Autodesk Fusion 360 part; units mm, degrees
note: some values were not read from the file. Set by a fixed rule: which face or edge a step refers to.
(part 2 of 3)
sketch "スケッチ1" plane through (0, 0, 0) normal (0, 0, 1) x (1, 0, 0)
  line L0 (95, 5) -> (-95, 5)
  line L1 (-95, 5) -> (-95, -5)
  line L2 (-95, -5) -> (95, -5)
  line L3 (95, -5) -> (95, 5)
  line L4 (95, 5) -> (-95, -5) construction
  line L5 (-95, 5) -> (95, -5) construction
  line L6 (90, 5) -> (-90, 5)
  line L7 (-90, 5) -> (-90, 25)
  line L8 (-90, 25) -> (90, 25)
  line L9 (90, 25) -> (90, 5)
  line L10 (90, 5) -> (-90, 25) construction
  line L11 (-90, 5) -> (90, 25) construction
  line L12 (90, 25) -> (-90, 25)
  line L13 (-90, 25) -> (-90, 45)
  line L14 (-90, 45) -> (90, 45)
  line L15 (90, 45) -> (90, 25)
  line L16 (90, 25) -> (-90, 45) construction
  line L17 (-90, 25) -> (90, 45) construction
  line L18 (40, -18) -> (-40, -18)
  line L19 (-40, -18) -> (-40, -5)
  line L20 (-40, -5) -> (40, -5)
  line L21 (40, -5) -> (40, -18)
  line L22 (40, -18) -> (-40, -5) construction
  line L23 (-40, -18) -> (40, -5) construction
  point P0 (0, 15)
  point P1 (0, 35)
  point P2 (0, -11.5)
  dimension "d1" = 190
  dimension "d2" = 10
  dimension "d3" = 20
  dimension "d4" = 180
  dimension "d5" = 180
  dimension "d6" = 20
  dimension "d9" = 13
  dimension "d10" = 80
  constraint horizontal L0
  constraint perpendicular L0 L1
  constraint parallel L0 L2
  constraint parallel L1 L3
  constraint coincident L4 origin
  constraint coincident L5 origin
  constraint horizontal L6
  constraint perpendicular L6 L7
  constraint parallel L6 L8
  constraint parallel L7 L9
  constraint coincident L10 P0
  constraint coincident L11 P0
  constraint vertical origin P0
  constraint coincident L0 L6.end
  constraint horizontal L12
  constraint perpendicular L12 L13
  constraint parallel L12 L14
  constraint parallel L13 L15
  constraint coincident L16 P1
  constraint coincident L17 P1
  constraint vertical origin P1
  constraint coincident L8 L7.end
  constraint horizontal L18
  constraint perpendicular L18 L19
  constraint parallel L18 L20
  constraint parallel L19 L21
  constraint coincident L22 P2
  constraint coincident L23 P2
  constraint vertical origin P2
  constraint coincident L2 L19.end
  measures "d1" distance of L1.end L2.end
  measures "d2" distance of L0.end L1.end
  measures "d3" distance of L6.end L7.end
  measures "d4" distance of L7.end L8.end
  measures "d5" distance of L13.end L14.end
  measures "d6" distance of L7.end L13.end
  measures "d9" distance of L18.end L19.end
  measures "d10" distance of L18.start L18.end
extrude "押し出し1" add sketch "スケッチ1" along normal blind 3
sketch "スケッチ2" plane through (0, 0, 0) normal (1, 0, 0) x (0, 1, 0)
  line L0 (-5, 0) -> (-18, 0)
  line L1 (-18, 0) -> (-18, 3)
  line L2 (-18, 3) -> (-5, 3)
  line L3 (-5, 3) -> (-5, 0)
  line L4 (5, 0) -> (-5, 0)
  line L5 (-5, 0) -> (-5, 3)
  line L6 (-5, 3) -> (5, 3)
  line L7 (5, 3) -> (5, 0)
  line L8 (45, 0) -> (5, 0)
  line L9 (5, 0) -> (5, 3)
  line L10 (5, 3) -> (45, 3)
  line L11 (45, 3) -> (45, 0)
  circle A0 centre (-22, 0) radius 2.5
  line L12 (-18, 0) -> (-18, 3)
  line L13 (-18, 0) -> (-19.5, 0)
  line L14 (-18, 3) -> (-24.5, 3)
  line L15 (-24.5, 0) -> (-24.5, 3)
  dimension "d11" = 5
  dimension "d12" = 4
  constraint coincident L0.end L1.start
  constraint coincident A0 L13.end
  constraint perpendicular L1 L13
  constraint coincident L1.end L2.start
  constraint perpendicular L12 L14
  constraint coincident A0 L15.start
  constraint perpendicular L14 L15
  constraint coincident L14.end L15.end
  measures "d11" diameter of A0
  measures "d12" distance of A0.centre L12
extrude "押し出し2" add sketch "スケッチ2" along normal mid plane 80 contours L1 A0 L12 L13 L14 L15 | A0
extrude "押し出し3" add sketch "スケッチ2" along normal mid plane 88 contours A0

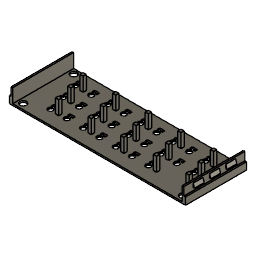
design "Keybord-Base-mid"
Autodesk Fusion 360 part; units mm, degrees
sketch "スケッチ1" plane through (0, 0, 0) normal (0, 0, 1) x (1, 0, 0)
  line L0 (108, 37.5) -> (-108, 37.5)
  line L1 (-108, 37.5) -> (-108, -37.5)
  line L2 (-108, -37.5) -> (108, -37.5)
  line L3 (108, -37.5) -> (108, 37.5)
  line L4 (108, 37.5) -> (-108, -37.5) construction
  line L5 (-108, 37.5) -> (108, -37.5) construction
  line L6 (-3.85, 21.5) -> (-3.85, 24)
  line L7 (-2, 27) -> (-2, 24)
  line L8 (-8, 27) -> (-2, 27)
  line L9 (-2, 24) -> (-8, 24)
  circle A0 centre (-5, 20) radius 2.65
  line L10 (-8, 24) -> (-8, 27)
  line L11 (-6.15, 24) -> (-6.15, 21.5)
  line L12 (-6.15, 21.5) -> (-3.85, 21.5)
  line L13 (-8, 24) -> (-2, 27) construction
  line L14 (-2, 24) -> (-8, 27) construction
  line L15 (-5, 20) -> (-5, 34)
  line L16 (-85, 20) -> (-85, 34)
  line L17 (-88, 24) -> (-88, 27)
  line L18 (-83.85, 21.5) -> (-83.85, 24)
  line L19 (-88, 24) -> (-82, 27) construction
  line L20 (-82, 27) -> (-82, 24)
  line L21 (-88, 27) -> (-82, 27)
  line L22 (-82, 24) -> (-88, 27) construction
  circle A1 centre (-85, 20) radius 2.65
  line L23 (-86.15, 24) -> (-86.15, 21.5)
  line L24 (-86.15, 21.5) -> (-83.85, 21.5)
  line L25 (-82, 24) -> (-88, 24)
  line L26 (-65, 20) -> (-65, 34)
  line L27 (-68, 24) -> (-68, 27)
  line L28 (-63.85, 21.5) -> (-63.85, 24)
  line L29 (-68, 24) -> (-62, 27) construction
  line L30 (-62, 27) -> (-62, 24)
  line L31 (-68, 27) -> (-62, 27)
  line L32 (-62, 24) -> (-68, 27) construction
  circle A2 centre (-65, 20) radius 2.65
  line L33 (-66.15, 24) -> (-66.15, 21.5)
  line L34 (-66.15, 21.5) -> (-63.85, 21.5)
  line L35 (-62, 24) -> (-68, 24)
  line L36 (-45, 20) -> (-45, 34)
  line L37 (-48, 24) -> (-48, 27)
  line L38 (-43.85, 21.5) -> (-43.85, 24)
  line L39 (-48, 24) -> (-42, 27) construction
  line L40 (-42, 27) -> (-42, 24)
  line L41 (-48, 27) -> (-42, 27)
  line L42 (-42, 24) -> (-48, 27) construction
  circle A3 centre (-45, 20) radius 2.65
  line L43 (-46.15, 24) -> (-46.15, 21.5)
  line L44 (-46.15, 21.5) -> (-43.85, 21.5)
  line L45 (-42, 24) -> (-48, 24)
  line L46 (-25, 20) -> (-25, 34)
  line L47 (-28, 24) -> (-28, 27)
  line L48 (-23.85, 21.5) -> (-23.85, 24)
  line L49 (-28, 24) -> (-22, 27) construction
  line L50 (-22, 27) -> (-22, 24)
  line L51 (-28, 27) -> (-22, 27)
  line L52 (-22, 24) -> (-28, 27) construction
  circle A4 centre (-25, 20) radius 2.65
  line L53 (-26.15, 24) -> (-26.15, 21.5)
  line L54 (-26.15, 21.5) -> (-23.85, 21.5)
  line L55 (-22, 24) -> (-28, 24)
  line L56 (15, 20) -> (15, 34)
  line L57 (12, 24) -> (12, 27)
  line L58 (16.15, 21.5) -> (16.15, 24)
  line L59 (12, 24) -> (18, 27) construction
  line L60 (18, 27) -> (18, 24)
  line L61 (12, 27) -> (18, 27)
  line L62 (18, 24) -> (12, 27) construction
  circle A5 centre (15, 20) radius 2.65
  line L63 (13.85, 24) -> (13.85, 21.5)
  line L64 (13.85, 21.5) -> (16.15, 21.5)
  line L65 (18, 24) -> (12, 24)
  line L66 (35, 20) -> (35, 34)
  line L67 (32, 24) -> (32, 27)
  line L68 (36.15, 21.5) -> (36.15, 24)
  line L69 (32, 24) -> (38, 27) construction
  line L70 (38, 27) -> (38, 24)
  line L71 (32, 27) -> (38, 27)
  line L72 (38, 24) -> (32, 27) construction
  circle A6 centre (35, 20) radius 2.65
  line L73 (33.85, 24) -> (33.85, 21.5)
  line L74 (33.85, 21.5) -> (36.15, 21.5)
  line L75 (38, 24) -> (32, 24)
  line L76 (55, 20) -> (55, 34)
  line L77 (52, 24) -> (52, 27)
  line L78 (56.15, 21.5) -> (56.15, 24)
  line L79 (52, 24) -> (58, 27) construction
  line L80 (58, 27) -> (58, 24)
  line L81 (52, 27) -> (58, 27)
  line L82 (58, 24) -> (52, 27) construction
  circle A7 centre (55, 20) radius 2.65
  line L83 (53.85, 24) -> (53.85, 21.5)
  line L84 (53.85, 21.5) -> (56.15, 21.5)
  line L85 (58, 24) -> (52, 24)
  line L86 (75, 20) -> (75, 34)
  line L87 (72, 24) -> (72, 27)
  line L88 (76.15, 21.5) -> (76.15, 24)
  line L89 (72, 24) -> (78, 27) construction
  line L90 (78, 27) -> (78, 24)
  line L91 (72, 27) -> (78, 27)
  line L92 (78, 24) -> (72, 27) construction
  circle A8 centre (75, 20) radius 2.65
  line L93 (73.85, 24) -> (73.85, 21.5)
  line L94 (73.85, 21.5) -> (76.15, 21.5)
  line L95 (78, 24) -> (72, 24)
  line L96 (95, 20) -> (95, 34)
  line L97 (92, 24) -> (92, 27)
  line L98 (96.15, 21.5) -> (96.15, 24)
  line L99 (92, 24) -> (98, 27) construction
  line L100 (98, 27) -> (98, 24)
  line L101 (92, 27) -> (98, 27)
  line L102 (98, 24) -> (92, 27) construction
  circle A9 centre (95, 20) radius 2.65
  line L103 (93.85, 24) -> (93.85, 21.5)
  line L104 (93.85, 21.5) -> (96.15, 21.5)
  line L105 (98, 24) -> (92, 24)
  line L106 (-3, 4) -> (-3, 7)
  line L107 (0, 0) -> (0, 14)
  line L108 (1.15, 1.5) -> (1.15, 4)
  line L109 (-3, 7) -> (3, 7)
  line L110 (-1.15, 1.5) -> (1.15, 1.5)
  line L111 (3, 7) -> (3, 4)
  line L112 (-3, 4) -> (3, 7) construction
  circle A10 centre (0, 0) radius 2.65
  line L113 (3, 4) -> (-3, 7) construction
  line L114 (3, 4) -> (-3, 4)
  line L115 (-1.15, 4) -> (-1.15, 1.5)
  circle A11 centre (-80, 0) radius 2.65
  line L116 (-83, 4) -> (-83, 7)
  line L117 (-83, 7) -> (-77, 7)
  line L118 (-77, 4) -> (-83, 4)
  line L119 (-77, 7) -> (-77, 4)
  line L120 (-82.2732, 4.8091) -> (-76.2732, 7.8091) construction
  line L121 (-76.2732, 4.8091) -> (-82.2732, 7.8091) construction
  line L122 (-81.15, 4) -> (-81.15, 1.5)
  line L123 (-81.15, 1.5) -> (-78.85, 1.5)
  line L124 (-78.85, 1.5) -> (-78.85, 4)
  circle A12 centre (-60, 0) radius 2.65
  line L125 (-63, 4) -> (-63, 7)
  line L126 (-63, 7) -> (-57, 7)
  line L127 (-57, 4) -> (-63, 4)
  line L128 (-57, 7) -> (-57, 4)
  line L129 (-62.2732, 4.8091) -> (-56.2732, 7.8091) construction
  line L130 (-56.2732, 4.8091) -> (-62.2732, 7.8091) construction
  line L131 (-61.15, 4) -> (-61.15, 1.5)
  line L132 (-61.15, 1.5) -> (-58.85, 1.5)
  line L133 (-58.85, 1.5) -> (-58.85, 4)
  circle A13 centre (-40, 0) radius 2.65
  line L134 (-43, 4) -> (-43, 7)
  line L135 (-43, 7) -> (-37, 7)
  line L136 (-37, 4) -> (-43, 4)
  line L137 (-37, 7) -> (-37, 4)
  line L138 (-42.2732, 4.8091) -> (-36.2732, 7.8091) construction
  line L139 (-36.2732, 4.8091) -> (-42.2732, 7.8091) construction
  line L140 (-41.15, 4) -> (-41.15, 1.5)
  line L141 (-41.15, 1.5) -> (-38.85, 1.5)
  line L142 (-38.85, 1.5) -> (-38.85, 4)
  circle A14 centre (-20, 0) radius 2.65
  line L143 (-23, 4) -> (-23, 7)
  line L144 (-23, 7) -> (-17, 7)
  line L145 (-17, 4) -> (-23, 4)
  line L146 (-17, 7) -> (-17, 4)
  line L147 (-22.2732, 4.8091) -> (-16.2732, 7.8091) construction
  line L148 (-16.2732, 4.8091) -> (-22.2732, 7.8091) construction
  line L149 (-21.15, 4) -> (-21.15, 1.5)
  line L150 (-21.15, 1.5) -> (-18.85, 1.5)
  line L151 (-18.85, 1.5) -> (-18.85, 4)
  circle A15 centre (20, 0) radius 2.65
  line L152 (17, 4) -> (17, 7)
  line L153 (17, 7) -> (23, 7)
  line L154 (23, 4) -> (17, 4)
  line L155 (23, 7) -> (23, 4)
  line L156 (17.7268, 4.8091) -> (23.7268, 7.8091) construction
  line L157 (23.7268, 4.8091) -> (17.7268, 7.8091) construction
  line L158 (18.85, 4) -> (18.85, 1.5)
  line L159 (18.85, 1.5) -> (21.15, 1.5)
  line L160 (21.15, 1.5) -> (21.15, 4)
  circle A16 centre (40, 0) radius 2.65
  line L161 (37, 4) -> (37, 7)
  line L162 (37, 7) -> (43, 7)
  line L163 (43, 4) -> (37, 4)
  line L164 (43, 7) -> (43, 4)
  line L165 (37.7268, 4.8091) -> (43.7268, 7.8091) construction
  line L166 (43.7268, 4.8091) -> (37.7268, 7.8091) construction
  line L167 (38.85, 4) -> (38.85, 1.5)
  line L168 (38.85, 1.5) -> (41.15, 1.5)
  line L169 (41.15, 1.5) -> (41.15, 4)
  circle A17 centre (60, 0) radius 2.65
  line L170 (57, 4) -> (57, 7)
  line L171 (57, 7) -> (63, 7)
  line L172 (63, 4) -> (57, 4)
  line L173 (63, 7) -> (63, 4)
  line L174 (57.7268, 4.8091) -> (63.7268, 7.8091) construction
  line L175 (63.7268, 4.8091) -> (57.7268, 7.8091) construction
  line L176 (58.85, 4) -> (58.85, 1.5)
  line L177 (58.85, 1.5) -> (61.15, 1.5)
  line L178 (61.15, 1.5) -> (61.15, 4)
  circle A18 centre (80, 0) radius 2.65
  line L179 (77, 4) -> (77, 7)
  line L180 (77, 7) -> (83, 7)
  line L181 (83, 4) -> (77, 4)
  line L182 (83, 7) -> (83, 4)
  line L183 (77.7268, 4.8091) -> (83.7268, 7.8091) construction
  line L184 (83.7268, 4.8091) -> (77.7268, 7.8091) construction
  line L185 (78.85, 4) -> (78.85, 1.5)
  line L186 (78.85, 1.5) -> (81.15, 1.5)
  line L187 (81.15, 1.5) -> (81.15, 4)
  line L188 (8, -16) -> (2, -13) construction
  line L189 (5, -20) -> (5, -6)
  line L190 (3.85, -18.5) -> (6.15, -18.5)
  line L191 (2, -13) -> (8, -13)
  line L192 (2, -16) -> (2, -13)
  line L193 (2, -16) -> (8, -13) construction
  line L194 (8, -13) -> (8, -16)
  circle A19 centre (5, -20) radius 2.65
  line L195 (3.85, -16) -> (3.85, -18.5)
  line L196 (6.15, -18.5) -> (6.15, -16)
  line L197 (8, -16) -> (2, -16)
  circle A20 centre (45, -20) radius 2.65
  line L198 (45, -20) -> (45, -6)
  line L199 (46.15, -18.5) -> (46.15, -16)
  line L200 (43.85, -18.5) -> (46.15, -18.5)
  line L201 (48, -16) -> (42, -16)
  line L202 (43.85, -16) -> (43.85, -18.5)
  line L203 (48, -16) -> (42, -13) construction
  line L204 (42, -16) -> (48, -13) construction
  line L205 (42, -13) -> (48, -13)
  line L206 (42, -16) -> (42, -13)
  line L207 (48, -13) -> (48, -16)
  circle A21 centre (25, -20) radius 2.65
  line L208 (25, -20) -> (25, -6)
  line L209 (26.15, -18.5) -> (26.15, -16)
  line L210 (23.85, -18.5) -> (26.15, -18.5)
  line L211 (28, -16) -> (22, -16)
  line L212 (23.85, -16) -> (23.85, -18.5)
  line L213 (28, -16) -> (22, -13) construction
  line L214 (22, -16) -> (28, -13) construction
  line L215 (22, -13) -> (28, -13)
  line L216 (22, -16) -> (22, -13)
  line L217 (28, -13) -> (28, -16)
  circle A22 centre (-15, -20) radius 2.65
  line L218 (-15, -20) -> (-15, -6)
  line L219 (-13.85, -18.5) -> (-13.85, -16)
  line L220 (-16.15, -18.5) -> (-13.85, -18.5)
  line L221 (-12, -16) -> (-18, -16)
  line L222 (-16.15, -16) -> (-16.15, -18.5)
  line L223 (-12, -16) -> (-18, -13) construction
  line L224 (-18, -16) -> (-12, -13) construction
  line L225 (-18, -13) -> (-12, -13)
  line L226 (-18, -16) -> (-18, -13)
  line L227 (-12, -13) -> (-12, -16)
  circle A23 centre (-35, -20) radius 2.65
  line L228 (-35, -20) -> (-35, -6)
  line L229 (-33.85, -18.5) -> (-33.85, -16)
  line L230 (-36.15, -18.5) -> (-33.85, -18.5)
  line L231 (-32, -16) -> (-38, -16)
  line L232 (-36.15, -16) -> (-36.15, -18.5)
  line L233 (-32, -16) -> (-38, -13) construction
  line L234 (-38, -16) -> (-32, -13) construction
  line L235 (-38, -13) -> (-32, -13)
  line L236 (-38, -16) -> (-38, -13)
  line L237 (-32, -13) -> (-32, -16)
  circle A24 centre (-55, -20) radius 2.65
  line L238 (-55, -20) -> (-55, -6)
  line L239 (-53.85, -18.5) -> (-53.85, -16)
  line L240 (-56.15, -18.5) -> (-53.85, -18.5)
  line L241 (-52, -16) -> (-58, -16)
  line L242 (-56.15, -16) -> (-56.15, -18.5)
  line L243 (-52, -16) -> (-58, -13) construction
  line L244 (-58, -16) -> (-52, -13) construction
  line L245 (-58, -13) -> (-52, -13)
  line L246 (-58, -16) -> (-58, -13)
  line L247 (-52, -13) -> (-52, -16)
  circle A25 centre (-75, -20) radius 2.65
  line L248 (-75, -20) -> (-75, -6)
  line L249 (-73.85, -18.5) -> (-73.85, -16)
  line L250 (-76.15, -18.5) -> (-73.85, -18.5)
  line L251 (-72, -16) -> (-78, -16)
  line L252 (-76.15, -16) -> (-76.15, -18.5)
  line L253 (-72, -16) -> (-78, -13) construction
  line L254 (-78, -16) -> (-72, -13) construction
  line L255 (-78, -13) -> (-72, -13)
  line L256 (-78, -16) -> (-78, -13)
  line L257 (-72, -13) -> (-72, -16)
  point P0 (0, 2.65)
  point P1 (-5, 25.5)
  point P2 (-5, 20)
  point P3 (-5, 20)
  point P4 (-5, 22.65)
  point P5 (-85, 22.65)
  point P6 (-85, 25.5)
  point P7 (-85, 20)
  point P8 (-85, 20)
  point P9 (-65, 22.65)
  point P10 (-65, 25.5)
  point P11 (-65, 20)
  point P12 (-65, 20)
  point P13 (-45, 22.65)
  point P14 (-45, 25.5)
  point P15 (-45, 20)
  point P16 (-45, 20)
  point P17 (-25, 22.65)
  point P18 (-25, 25.5)
  point P19 (-25, 20)
  point P20 (-25, 20)
  point P21 (15, 22.65)
  point P22 (15, 25.5)
  point P23 (15, 20)
  point P24 (15, 20)
  point P25 (35, 22.65)
  point P26 (35, 25.5)
  point P27 (35, 20)
  point P28 (35, 20)
  point P29 (55, 22.65)
  point P30 (55, 25.5)
  point P31 (55, 20)
  point P32 (55, 20)
  point P33 (75, 22.65)
  point P34 (75, 25.5)
  point P35 (75, 20)
  point P36 (75, 20)
  point P37 (95, 22.65)
  point P38 (95, 25.5)
  point P39 (95, 20)
  point P40 (95, 20)
  point P41 (-10.2565, 1.2142)
  point P42 (-10.2565, 1.2142)
  point P43 (0, 5.5)
  point P44 (0, 2.65)
  point P45 (5, -20)
  point P46 (5, -17.35)
  point P47 (5, -14.5)
  point P48 (5, -20)
  point P49 (45, -17.35)
  point P50 (45, -20)
  point P51 (45, -20)
  point P52 (45, -14.5)
  point P53 (25, -17.35)
  point P54 (25, -20)
  point P55 (25, -20)
  point P56 (25, -14.5)
  point P57 (-15, -17.35)
  point P58 (-15, -20)
  point P59 (-15, -20)
  point P60 (-15, -14.5)
  point P61 (-35, -17.35)
  point P62 (-35, -20)
  point P63 (-35, -20)
  point P64 (-35, -14.5)
  point P65 (-55, -17.35)
  point P66 (-55, -20)
  point P67 (-55, -20)
  point P68 (-55, -14.5)
  point P69 (-75, -17.35)
  point P70 (-75, -20)
  point P71 (-75, -20)
  point P72 (-75, -14.5)
  dimension "d1" = 216
  dimension "d2" = 75
  dimension "d85" = 5.3
  dimension "d86" = 2.3
  dimension "d87" = 6
  dimension "d88" = 3
  dimension "d89" = 5.5
  dimension "d90" = 1.5
  dimension "d92" = 20
  dimension "d94" = 2.3
  dimension "d97" = 20
  dimension "d98" = 0
  dimension "d99" = 5
  dimension "d114" = 5.3
  dimension "d115" = 2.3
  dimension "d116" = 6
  dimension "d117" = 3
  dimension "d118" = 5.5
  dimension "d119" = 1.5
  dimension "d120" = 2.3
  dimension "d138" = 5.3
  dimension "d139" = 2.3
  dimension "d140" = 6
  dimension "d141" = 3
  dimension "d142" = 5.5
  dimension "d143" = 1.5
  dimension "d144" = 2.3
  dimension "d145" = 5
  dimension "d146" = 20
  dimension "d149" = -20
  dimension "d150" = 0
  constraint horizontal L0
  constraint perpendicular L0 L1
  constraint parallel L0 L2
  constraint parallel L1 L3
  constraint coincident L4 L107.start
  constraint coincident L5 L107.start
  constraint coincident L107.start A10.centre
  constraint vertical L107.start P44
  constraint coincident P3 P2
  constraint parallel L6 L11
  constraint coincident P4 A0
  constraint vertical P3 P4
  constraint horizontal L9
  constraint perpendicular L9 L10
  constraint parallel L8 L9
  constraint parallel L7 L10
  constraint coincident P1 L14
  constraint coincident P1 L13
  constraint perpendicular L11 L12
  constraint coincident L11.start L9
  constraint coincident L6.end L9
  constraint perpendicular L8 L15
  constraint midpoint L8 L15
  constraint coincident P42 P41
  constraint parallel L108 L115
  constraint coincident P44 A10
  constraint horizontal L114
  constraint perpendicular L106 L114
  constraint parallel L109 L114
  constraint parallel L106 L111
  constraint coincident P43 L113
  constraint coincident P43 L112
  constraint perpendicular L110 L115
  constraint coincident L115.start L114
  constraint coincident L108.end L114
  constraint perpendicular L107 L109
  constraint midpoint L107 L109
  constraint coincident P48 P45
  constraint parallel L195 L196
  constraint coincident P46 A19
  constraint vertical P48 P46
  constraint horizontal L197
  constraint perpendicular L192 L197
  constraint parallel L191 L197
  constraint parallel L192 L194
  constraint coincident P47 L188
  constraint coincident P47 L193
  constraint perpendicular L190 L195
  constraint coincident L195.start L197
  constraint coincident L196.end L197
  constraint perpendicular L189 L191
  constraint midpoint L189 L191
  measures "d1" distance of L1.end L2.end
  measures "d2" distance of L0.end L1.end
  measures "d85" diameter of A0
  measures "d86" distance of L11.end L6.start
  measures "d87" distance of L7.start L8.start
  measures "d88" distance of L9.end L8.start
  measures "d89" distance of P1 P3
  measures "d90" distance of P3 L12
  measures "d92" vertical distance of L107.start P3
  measures "d99" horizontal distance of L107.start P3
  measures "d114" diameter of A10
  measures "d115" distance of L110.start L108.start
  measures "d116" distance of L106.end L109.end
  measures "d117" distance of L106.end L106.start
  measures "d118" distance of P43 L107.start
  measures "d119" distance of L107.start L110
  measures "d138" diameter of A19
  measures "d139" distance of L190.start L190.end
  measures "d140" distance of L188.end L191.end
  measures "d141" distance of L188.end L192.start
  measures "d142" distance of P48 P47
  measures "d143" distance of P48 L190
  measures "d145" horizontal distance of L107.start P48
  measures "d146" vertical distance of L107.start P48
extrude "押し出し1" add sketch "スケッチ1" along normal blind 2
fillet "フィレット1" radius 0.5 52 faces at (94.3639, 17.4275, 1.3333) (97.1025, 21.6131, 1.3333) (74.3639, 17.4275, 1.3333) (77.1025, 21.6131, 1.3333) (57.6468, 19.8702, 1.3333) (57.1025, 21.6131, 1.3333) (37.6468, 19.8702, 1.3333) (37.1025, 21.6131, 1.3333) (17.6468, 19.8702, 1.3333) (16.2603, 22.3311, 1.3333) (-2.3532, 19.8702, 1.3333) (-3.7397, 22.3311, 1.3333) (21.5738, 2.1321, 1.3333) (22.6468, -0.1298, 1.3333) (-22.3532, 19.8702, 1.3333) (-22.5332, 20.9681, 1.3333) (-42.3532, 19.8702, 1.3333) (-42.8975, 21.6131, 1.3333) (-65.6361, 17.4275, 1.3333) (-62.8975, 21.6131, 1.3333) (-85.6361, 17.4275, 1.3333) (-82.8975, 21.6131, 1.3333) (-78.6321, 2.2697, 1.3333) (-80.6361, -2.5725, 1.3333) (-58.4262, 2.1321, 1.3333) (-57.3532, -0.1298, 1.3333) (-38.4262, 2.1321, 1.3333) (-37.3532, -0.1298, 1.3333) (-18.1437, 1.8912, 1.3333) (-17.3532, -0.1298, 1.3333) (2.6468, -0.1298, 1.3333) (1.2603, 2.3311, 1.3333) (7.6468, -20.1298, 1.3333) (7.4668, -19.0319, 1.3333) (-12.5332, -19.0319, 1.3333) (-12.3532, -20.1298, 1.3333) (-32.8975, -18.3869, 1.3333) (-32.3532, -20.1298, 1.3333) (-72.8975, -18.3869, 1.3333) (-75.6361, -22.5725, 1.3333) (-52.8975, -18.3869, 1.3333) (-52.3532, -20.1298, 1.3333) (41.5738, 2.1321, 1.3333) (42.6468, -0.1298, 1.3333) (27.4668, -19.0319, 1.3333) (27.6468, -20.1298, 1.3333) (47.1025, -18.3869, 1.3333) (47.6468, -20.1298, 1.3333) (61.5738, 2.1321, 1.3333) (62.6468, -0.1298, 1.3333) (81.3679, 2.2697, 1.3333) (79.3639, -2.5725, 1.3333)
sketch "スケッチ2" plane through (0, 0, 2) normal (0, 0, 1) x (-1, 0, 0)
  line L0 (-108, 37.5) -> (-108, -37.5)
  line L1 (-108, -37.5) -> (108, -37.5)
  line L2 (108, -37.5) -> (108, 37.5)
  line L3 (108, 37.5) -> (-108, 37.5)
  line L4 (108, -37.5) -> (104, -37.5)
  line L5 (104, -37.5) -> (104, 37.5)
  line L6 (104, 37.5) -> (108, 37.5)
  line L7 (108, 37.5) -> (108, -37.5)
  line L8 (-108, -37.5) -> (-104, -37.5)
  line L9 (-104, -37.5) -> (-104, 37.5)
  line L10 (-104, 37.5) -> (-108, 37.5)
  line L11 (-108, 37.5) -> (-108, -37.5)
  line L12 (-18.85, -2.9326) -> (-18.85, -4)
  line L13 (-18.85, -4) -> (-17, -4)
  line L14 (-17, -4) -> (-17, -7)
  line L15 (-17, -7) -> (-23, -7)
  line L16 (-23, -7) -> (-23, -4)
  line L17 (-23, -4) -> (-21.15, -4)
  line L18 (-21.15, -4) -> (-21.15, -2.9326)
  line L19 (16.15, 17.0674) -> (16.15, 16)
  line L20 (16.15, 16) -> (18, 16)
  line L21 (18, 16) -> (18, 13)
  line L22 (18, 13) -> (12, 13)
  line L23 (12, 13) -> (12, 16)
  line L24 (12, 16) -> (13.85, 16)
  line L25 (13.85, 16) -> (13.85, 17.0674)
  line L26 (76.15, 17.0674) -> (76.15, 16)
  line L27 (76.15, 16) -> (78, 16)
  line L28 (78, 16) -> (78, 13)
  line L29 (78, 13) -> (72, 13)
  line L30 (72, 13) -> (72, 16)
  line L31 (72, 16) -> (73.85, 16)
  line L32 (73.85, 16) -> (73.85, 17.0674)
  line L33 (-38.85, -2.9326) -> (-38.85, -4)
  line L34 (-38.85, -4) -> (-37, -4)
  line L35 (-37, -4) -> (-37, -7)
  line L36 (-37, -7) -> (-43, -7)
  line L37 (-43, -7) -> (-43, -4)
  line L38 (-43, -4) -> (-41.15, -4)
  line L39 (-41.15, -4) -> (-41.15, -2.9326)
  line L40 (-43.85, 17.0674) -> (-43.85, 16)
  line L41 (-43.85, 16) -> (-42, 16)
  line L42 (-42, 16) -> (-42, 13)
  line L43 (-42, 13) -> (-48, 13)
  line L44 (-48, 13) -> (-48, 16)
  line L45 (-48, 16) -> (-46.15, 16)
  line L46 (-46.15, 16) -> (-46.15, 17.0674)
  line L47 (-23.85, 17.0674) -> (-23.85, 16)
  line L48 (-23.85, 16) -> (-22, 16)
  line L49 (-22, 16) -> (-22, 13)
  line L50 (-22, 13) -> (-28, 13)
  line L51 (-28, 13) -> (-28, 16)
  line L52 (-28, 16) -> (-26.15, 16)
  line L53 (-26.15, 16) -> (-26.15, 17.0674)
  line L54 (1.15, -4) -> (3, -4)
  line L55 (3, -4) -> (3, -7)
  line L56 (3, -7) -> (-3, -7)
  line L57 (-3, -7) -> (-3, -4)
  line L58 (-3, -4) -> (-1.15, -4)
  line L59 (-1.15, -4) -> (-1.15, -2.9326)
  line L60 (1.15, -2.9326) -> (1.15, -4)
  line L61 (61.15, -2.9326) -> (61.15, -4)
  line L62 (61.15, -4) -> (63, -4)
  line L63 (63, -4) -> (63, -7)
  line L64 (63, -7) -> (57, -7)
  line L65 (57, -7) -> (57, -4)
  line L66 (57, -4) -> (58.85, -4)
  line L67 (58.85, -4) -> (58.85, -2.9326)
  line L68 (56.15, 17.0674) -> (56.15, 16)
  line L69 (56.15, 16) -> (58, 16)
  line L70 (58, 16) -> (58, 13)
  line L71 (58, 13) -> (52, 13)
  line L72 (52, 13) -> (52, 16)
  line L73 (52, 16) -> (53.85, 16)
  line L74 (53.85, 16) -> (53.85, 17.0674)
  line L75 (36.15, 17.0674) -> (36.15, 16)
  line L76 (36.15, 16) -> (38, 16)
  line L77 (38, 16) -> (38, 13)
  line L78 (38, 13) -> (32, 13)
  line L79 (32, 13) -> (32, 16)
  line L80 (32, 16) -> (33.85, 16)
  line L81 (33.85, 16) -> (33.85, 17.0674)
  line L82 (-3.85, 17.0674) -> (-3.85, 16)
  line L83 (-3.85, 16) -> (-2, 16)
  line L84 (-2, 16) -> (-2, 13)
  line L85 (-2, 13) -> (-8, 13)
  line L86 (-8, 13) -> (-8, 16)
  line L87 (-8, 16) -> (-6.15, 16)
  line L88 (-6.15, 16) -> (-6.15, 17.0674)
  line L89 (-58.85, -2.9326) -> (-58.85, -4)
  line L90 (-58.85, -4) -> (-57, -4)
  line L91 (-57, -4) -> (-57, -7)
  line L92 (-57, -7) -> (-63, -7)
  line L93 (-63, -7) -> (-63, -4)
  line L94 (-63, -4) -> (-61.15, -4)
  line L95 (-61.15, -4) -> (-61.15, -2.9326)
  line L96 (81.15, -2.9326) -> (81.15, -4)
  line L97 (81.15, -4) -> (83, -4)
  line L98 (83, -4) -> (83, -7)
  line L99 (83, -7) -> (77, -7)
  line L100 (77, -7) -> (77, -4)
  line L101 (77, -4) -> (78.85, -4)
  line L102 (78.85, -4) -> (78.85, -2.9326)
  line L103 (21.15, -2.9326) -> (21.15, -4)
  line L104 (21.15, -4) -> (23, -4)
  line L105 (23, -4) -> (23, -7)
  line L106 (23, -7) -> (17, -7)
  line L107 (17, -7) -> (17, -4)
  line L108 (17, -4) -> (18.85, -4)
  line L109 (18.85, -4) -> (18.85, -2.9326)
  line L110 (-78.85, -2.9326) -> (-78.85, -4)
  line L111 (-78.85, -4) -> (-77, -4)
  line L112 (-77, -4) -> (-77, -7)
  line L113 (-77, -7) -> (-83, -7)
  line L114 (-83, -7) -> (-83, -4)
  line L115 (-83, -4) -> (-81.15, -4)
  line L116 (-81.15, -4) -> (-81.15, -2.9326)
  line L117 (41.15, -2.9326) -> (41.15, -4)
  line L118 (41.15, -4) -> (43, -4)
  line L119 (43, -4) -> (43, -7)
  line L120 (43, -7) -> (37, -7)
  line L121 (37, -7) -> (37, -4)
  line L122 (37, -4) -> (38.85, -4)
  line L123 (38.85, -4) -> (38.85, -2.9326)
  line L124 (-93.85, -22.9326) -> (-93.85, -24)
  line L125 (-93.85, -24) -> (-92, -24)
  line L126 (-92, -24) -> (-92, -27)
  line L127 (-92, -27) -> (-98, -27)
  line L128 (-98, -27) -> (-98, -24)
  line L129 (-98, -24) -> (-96.15, -24)
  line L130 (-96.15, -24) -> (-96.15, -22.9326)
  line L131 (26.15, -22.9326) -> (26.15, -24)
  line L132 (26.15, -24) -> (28, -24)
  line L133 (28, -24) -> (28, -27)
  line L134 (28, -27) -> (22, -27)
  line L135 (22, -27) -> (22, -24)
  line L136 (22, -24) -> (23.85, -24)
  line L137 (23.85, -24) -> (23.85, -22.9326)
  line L138 (46.15, -22.9326) -> (46.15, -24)
  line L139 (46.15, -24) -> (48, -24)
  line L140 (48, -24) -> (48, -27)
  line L141 (48, -27) -> (42, -27)
  line L142 (42, -27) -> (42, -24)
  line L143 (42, -24) -> (43.85, -24)
  line L144 (43.85, -24) -> (43.85, -22.9326)
  line L145 (6.15, -24) -> (8, -24)
  line L146 (8, -24) -> (8, -27)
  line L147 (8, -27) -> (2, -27)
  line L148 (2, -27) -> (2, -24)
  line L149 (2, -24) -> (3.85, -24)
  line L150 (3.85, -24) -> (3.85, -22.9326)
  line L151 (6.15, -22.9326) -> (6.15, -24)
  line L152 (66.15, -22.9326) -> (66.15, -24)
  line L153 (66.15, -24) -> (68, -24)
  line L154 (68, -24) -> (68, -27)
  line L155 (68, -27) -> (62, -27)
  line L156 (62, -27) -> (62, -24)
  line L157 (62, -24) -> (63.85, -24)
  line L158 (63.85, -24) -> (63.85, -22.9326)
  line L159 (86.15, -22.9326) -> (86.15, -24)
  line L160 (86.15, -24) -> (88, -24)
  line L161 (88, -24) -> (88, -27)
  line L162 (88, -27) -> (82, -27)
  line L163 (82, -27) -> (82, -24)
  line L164 (82, -24) -> (83.85, -24)
  line L165 (83.85, -24) -> (83.85, -22.9326)
  line L166 (-13.85, -22.9326) -> (-13.85, -24)
  line L167 (-13.85, -24) -> (-12, -24)
  line L168 (-12, -24) -> (-12, -27)
  line L169 (-12, -27) -> (-18, -27)
  line L170 (-18, -27) -> (-18, -24)
  line L171 (-18, -24) -> (-16.15, -24)
  line L172 (-16.15, -24) -> (-16.15, -22.9326)
  line L173 (-53.85, -22.9326) -> (-53.85, -24)
  line L174 (-53.85, -24) -> (-52, -24)
  line L175 (-52, -24) -> (-52, -27)
  line L176 (-52, -27) -> (-58, -27)
  line L177 (-58, -27) -> (-58, -24)
  line L178 (-58, -24) -> (-56.15, -24)
  line L179 (-56.15, -24) -> (-56.15, -22.9326)
  line L180 (-33.85, -22.9326) -> (-33.85, -24)
  line L181 (-33.85, -24) -> (-32, -24)
  line L182 (-32, -24) -> (-32, -27)
  line L183 (-32, -27) -> (-38, -27)
  line L184 (-38, -27) -> (-38, -24)
  line L185 (-38, -24) -> (-36.15, -24)
  line L186 (-36.15, -24) -> (-36.15, -22.9326)
  line L187 (-73.85, -22.9326) -> (-73.85, -24)
  line L188 (-73.85, -24) -> (-72, -24)
  line L189 (-72, -24) -> (-72, -27)
  line L190 (-72, -27) -> (-78, -27)
  line L191 (-78, -27) -> (-78, -24)
  line L192 (-78, -24) -> (-76.15, -24)
  line L193 (-76.15, -24) -> (-76.15, -22.9326)
  arc A0 (-78.85, -2.9326) -> (-81.15, -2.9326) centre (-80, 0) ccw
  arc A1 (-58.85, -2.9326) -> (-61.15, -2.9326) centre (-60, 0) ccw
  arc A2 (-43.85, 17.0674) -> (-46.15, 17.0674) centre (-45, 20) ccw
  arc A3 (-23.85, 17.0674) -> (-26.15, 17.0674) centre (-25, 20) ccw
  arc A4 (-38.85, -2.9326) -> (-41.15, -2.9326) centre (-40, 0) ccw
  arc A5 (56.15, 17.0674) -> (53.85, 17.0674) centre (55, 20) ccw
  arc A6 (76.15, 17.0674) -> (73.85, 17.0674) centre (75, 20) ccw
  arc A7 (36.15, 17.0674) -> (33.85, 17.0674) centre (35, 20) ccw
  arc A8 (16.15, 17.0674) -> (13.85, 17.0674) centre (15, 20) ccw
  arc A9 (-3.85, 17.0674) -> (-6.15, 17.0674) centre (-5, 20) ccw
  arc A10 (1.15, -2.9326) -> (-1.15, -2.9326) centre (0, 0) ccw
  arc A11 (21.15, -2.9326) -> (18.85, -2.9326) centre (20, 0) ccw
  arc A12 (41.15, -2.9326) -> (38.85, -2.9326) centre (40, 0) ccw
  arc A13 (61.15, -2.9326) -> (58.85, -2.9326) centre (60, 0) ccw
  arc A14 (81.15, -2.9326) -> (78.85, -2.9326) centre (80, 0) ccw
  arc A15 (86.15, -22.9326) -> (83.85, -22.9326) centre (85, -20) ccw
  arc A16 (66.15, -22.9326) -> (63.85, -22.9326) centre (65, -20) ccw
  arc A17 (46.15, -22.9326) -> (43.85, -22.9326) centre (45, -20) ccw
  arc A18 (26.15, -22.9326) -> (23.85, -22.9326) centre (25, -20) ccw
  arc A19 (-18.85, -2.9326) -> (-21.15, -2.9326) centre (-20, 0) ccw
  arc A20 (6.15, -22.9326) -> (3.85, -22.9326) centre (5, -20) ccw
  arc A21 (-13.85, -22.9326) -> (-16.15, -22.9326) centre (-15, -20) ccw
  arc A22 (-33.85, -22.9326) -> (-36.15, -22.9326) centre (-35, -20) ccw
  arc A23 (-53.85, -22.9326) -> (-56.15, -22.9326) centre (-55, -20) ccw
  arc A24 (-73.85, -22.9326) -> (-76.15, -22.9326) centre (-75, -20) ccw
  arc A25 (-93.85, -22.9326) -> (-96.15, -22.9326) centre (-95, -20) ccw
  line L194 (77, -22) -> (73, -22)
  line L195 (73, -22) -> (73, -18)
  line L196 (73, -18) -> (77, -18)
  line L197 (77, -18) -> (77, -22)
  line L198 (37, -22) -> (33, -22)
  line L199 (33, -22) -> (33, -18)
  line L200 (37, -18) -> (37, -22)
  line L201 (33, -18) -> (37, -18)
  line L202 (-3, -22) -> (-7, -22)
  line L203 (-7, -22) -> (-7, -18)
  line L204 (-3, -18) -> (-3, -22)
  line L205 (-7, -18) -> (-3, -18)
  line L206 (-43, -22) -> (-47, -22)
  line L207 (-47, -22) -> (-47, -18)
  line L208 (-43, -18) -> (-43, -22)
  line L209 (-47, -18) -> (-43, -18)
  line L210 (-83, -22) -> (-87, -22)
  line L211 (-87, -22) -> (-87, -18)
  line L212 (-83, -18) -> (-83, -22)
  line L213 (-87, -18) -> (-83, -18)
  line L214 (72, -2) -> (68, -2)
  line L215 (68, -2) -> (68, 2)
  line L216 (68, 2) -> (72, 2)
  line L217 (72, 2) -> (72, -2)
  line L218 (67, 18) -> (63, 18)
  line L219 (63, 18) -> (63, 22)
  line L220 (63, 22) -> (67, 22)
  line L221 (67, 22) -> (67, 18)
  line L222 (32, -2) -> (28, -2)
  line L223 (28, -2) -> (28, 2)
  line L224 (28, 2) -> (32, 2)
  line L225 (32, 2) -> (32, -2)
  line L226 (-8, -2) -> (-12, -2)
  line L227 (-12, -2) -> (-12, 2)
  line L228 (-12, 2) -> (-8, 2)
  line L229 (-8, 2) -> (-8, -2)
  line L230 (-48, -2) -> (-52, -2)
  line L231 (-52, -2) -> (-52, 2)
  line L232 (-52, 2) -> (-48, 2)
  line L233 (-48, 2) -> (-48, -2)
  line L234 (-88, -2) -> (-92, -2)
  line L235 (-92, -2) -> (-92, 2)
  line L236 (-92, 2) -> (-88, 2)
  line L237 (-88, 2) -> (-88, -2)
  line L238 (27, 18) -> (23, 18)
  line L239 (23, 18) -> (23, 22)
  line L240 (23, 22) -> (27, 22)
  line L241 (27, 22) -> (27, 18)
  line L242 (-13, 18) -> (-17, 18)
  line L243 (-17, 18) -> (-17, 22)
  line L244 (-17, 22) -> (-13, 22)
  line L245 (-13, 22) -> (-13, 18)
  line L246 (-53, 18) -> (-57, 18)
  line L247 (-57, 18) -> (-57, 22)
  line L248 (-57, 22) -> (-53, 22)
  line L249 (-53, 22) -> (-53, 18)
  line L250 (-93, 18) -> (-97, 18)
  line L251 (-97, 18) -> (-97, 22)
  line L252 (-97, 22) -> (-93, 22)
  line L253 (-93, 22) -> (-93, 18)
  dimension "d55" = 4
  dimension "d56" = 4
  dimension "d153" = 5
  dimension "d154" = 5
  dimension "d155" = 4
  dimension "d156" = 5
  dimension "d159" = -40
  dimension "d160" = 0
  dimension "d161" = 5
  dimension "d162" = 5
  dimension "d163" = 4
  dimension "d164" = 5
  dimension "d165" = 5
  dimension "d166" = 5
  dimension "d167" = 5
  dimension "d168" = 4
  dimension "d171" = -40
  dimension "d172" = 0
  dimension "d175" = -40
  dimension "d176" = 0
  constraint horizontal L4
  constraint vertical L5
  constraint horizontal L6
  constraint vertical L7
  constraint coincident L1.end L2.start
  constraint horizontal L8
  constraint vertical L9
  constraint horizontal L10
  constraint vertical L11
  constraint coincident L3 L9.end
  constraint coincident L0.end L1.start
  constraint horizontal L194
  constraint vertical L195
  constraint horizontal L196
  constraint vertical L197
  constraint horizontal L214
  constraint vertical L215
  constraint horizontal L216
  constraint vertical L217
  constraint horizontal L218
  constraint vertical L219
  constraint horizontal L220
  constraint vertical L221
  measures "d55" distance of L1.end L4.end
  measures "d56" distance of L0.end L8.end
  measures "d153" distance of L163 L197
  measures "d154" distance of L154 L195
  measures "d155" distance of L194 L196
  measures "d156" distance of L162 L194
  measures "d161" distance of L100 L217
  measures "d162" distance of L63 L215
  measures "d163" distance of L214 L216
  measures "d164" distance of L99 L214
  measures "d165" distance of L29 L218
  measures "d166" distance of L30 L221
  measures "d167" distance of L70 L219
  measures "d168" distance of L218 L220
extrude "押し出し2" add sketch "スケッチ2" along normal blind 17 contours L0 L1 L3 L8 L9 L10 L11 | L1 L2 L3 L4 L5 L6 L7 | L194 L195 L196 L197 | L198 L199 L200 L201 | L202 L203 L204 L205 | L206 L207 L208 L209 | L210 L211 L212 L213 | L214 L215 L216 L217 | L218 L219 L220 L221 | L222 L223 L224 L225 | L226 L227 L228 L229 | L230 L231 L232 L233 | L234 L235 L236 L237 | L238 L239 L240 L241 | L242 L243 L244 L245 | L246 L247 L248 L249 | L250 L251 L252 L253
sketch "スケッチ3" plane through (0, 0, 19) normal (0, 0, 1) x (-1, 0, 0)
  line L0 (-108, 37.5) -> (-108, -37.5)
  line L1 (-108, -37.5) -> (-104, -37.5)
  line L2 (-104, -37.5) -> (-104, 37.5)
  line L3 (-104, 37.5) -> (-108, 37.5)
  line L4 (-108, -37.5) -> (-106, -37.5)
  line L5 (-106, -37.5) -> (-106, 37.5)
  line L6 (-106, 37.5) -> (-108, 37.5)
  line L7 (-108, 37.5) -> (-108, -37.5)
  line L8 (108, 37.5) -> (104, 37.5)
  line L9 (104, 37.5) -> (104, -37.5)
  line L10 (104, -37.5) -> (108, -37.5)
  line L11 (108, -37.5) -> (108, 37.5)
  line L12 (108, -37.5) -> (106, -37.5)
  line L13 (106, -37.5) -> (106, 37.5)
  line L14 (106, 37.5) -> (108, 37.5)
  line L15 (108, 37.5) -> (108, -37.5)
  constraint horizontal L4
  constraint vertical L5
  constraint horizontal L6
  constraint vertical L7
  constraint midpoint L3 L5.end
  constraint coincident L0.end L1.start
  constraint horizontal L12
  constraint vertical L13
  constraint horizontal L14
  constraint vertical L15
  constraint midpoint L8 L13.end
  constraint coincident L10.end L11.start
extrude "押し出し3" cut sketch "スケッチ3" against normal blind 10 contours L0 L1 L3 L4 L5 L6 L7 | L8 L10 L11 L12 L13 L14 L15
ref_plane "作業平面1" through (0, 20, 0) normal (0, 1, 0) x (0, 0, 1)
ref_plane "作業平面2" through (0, -20, 0) normal (0, 1, 0) x (0, 0, 1)
sketch "スケッチ5" plane through (0, 20, 0) normal (0, 1, 0) x (1, 0, 0)
  line L0 (-106, -17) -> (-106, -12.2)
  line L1 (-104, -19) -> (-106, -19)
  line L2 (0, -20) -> (0, -2.5)
  line L3 (-106, -12.2) -> (-107.5, -12.2)
  line L4 (-107.5, -12.2) -> (-106, -17)
  line L5 (-108, -9) -> (-106, -9)
  line L6 (-106, -9) -> (-106, -19)
  line L7 (-106, -19) -> (-104, -19)
  line L8 (-104, -19) -> (-104, -2)
  line L9 (-104, -2) -> (104, -2)
  line L10 (108, 0) -> (-108, 0)
  line L11 (-108, 0) -> (-108, -9)
  line L12 (104, -19) -> (104, -2)
  line L13 (108, 0) -> (108, -9)
  line L14 (106, -9) -> (106, -19)
  line L15 (108, -9) -> (106, -9)
  line L16 (106, -12.2) -> (107.5, -12.2)
  line L17 (106, -17) -> (106, -12.2)
  line L18 (107.5, -12.2) -> (106, -17)
  line L19 (106, -19) -> (104, -19)
  line L20 (104, -19) -> (106, -19)
  dimension "d68" = 1.5
  dimension "d69" = 4.8
  dimension "d70" = 2
  constraint perpendicular L0 L3
  constraint vertical L0
  constraint collinear L0 L6
  constraint symmetric L0.end L2 L16.start
  constraint symmetric L0.start L2 L17.start
  constraint symmetric L1.start L2 L12.start
  constraint symmetric L1.end L2 L14.end
  constraint symmetric L2 L3.end L16.end
  constraint symmetric L2 L5.start L13.end
  constraint symmetric L2 L5.end L14.start
  constraint symmetric L2 L1.end L14.end
  constraint symmetric L2 L1.start L12.start
  constraint symmetric L2 L8.end L9.end
  constraint symmetric L2 L10.end L10.start
  measures "d68" distance of L0.end L3.end
  measures "d69" distance of L0.end L0.start
  measures "d70" distance of L0.start L1
extrude "押し出し4" add sketch "スケッチ5" along normal mid plane 12 contours L0 L3 L4 L6 | L14 L16 L17 L18
sketch "スケッチ6" plane through (0, 0, 0) normal (0, 1, 0) x (1, 0, 0)
  line L0 (-106, -12.2) -> (-107.5, -12.2)
  line L1 (-106, -12.2) -> (-106, -17)
  line L2 (-106, -17) -> (-107.5, -12.2)
  line L3 (-106, -9) -> (-108, -9)
  line L4 (-108, -9) -> (-108, 0)
  line L5 (-108, 0) -> (108, 0)
  line L6 (108, 0) -> (108, -9)
  line L7 (108, -9) -> (106, -9)
  line L8 (106, -9) -> (106, -19)
  line L9 (106, -19) -> (104, -19)
  line L10 (104, -19) -> (104, -2)
  line L11 (104, -2) -> (-104, -2)
  line L12 (-104, -2) -> (-104, -19)
  line L13 (-104, -19) -> (-106, -19)
  line L14 (-106, -19) -> (-106, -9)
  line L15 (0, -20) -> (0, -2.5)
  line L16 (106, -12.2) -> (107.5, -12.2)
  line L17 (104, -19) -> (106, -19)
  line L18 (106, -12.2) -> (106, -17)
  line L19 (106, -19) -> (106, -9)
  line L20 (106, -17) -> (107.5, -12.2)
  line L21 (106, -9) -> (108, -9)
  dimension "d71" = 1.5
  dimension "d73" = 4.8
  dimension "d76" = 2
  constraint horizontal L0
  constraint perpendicular L0 L1
  constraint collinear L1 L14
  constraint symmetric L0.start L15 L16.start
  constraint symmetric L0.end L15 L16.end
  constraint symmetric L1.end L15 L18.end
  constraint symmetric L3.start L15 L7.end
  constraint symmetric L3.end L15 L6.end
  constraint symmetric L12.end L15 L9.end
  constraint symmetric L13.end L15 L8.end
  measures "d71" distance of L0.start L0.end
  measures "d73" distance of L0 L1.end
  measures "d76" distance of L1.end L13
extrude "押し出し5" add sketch "スケッチ6" along normal mid plane 12 contours L0 L1 L2 L14 | L8 L16 L18 L19 L20
sketch "スケッチ7" plane through (0, -20, 0) normal (0, 1, 0) x (1, 0, 0)
  line L0 (-106, -9) -> (-108, -9)
  line L1 (-108, -9) -> (-108, 0)
  line L2 (-108, 0) -> (108, 0)
  line L3 (108, 0) -> (108, -9)
  line L4 (108, -9) -> (106, -9)
  line L5 (106, -9) -> (106, -19)
  line L6 (106, -19) -> (104, -19)
  line L7 (104, -19) -> (104, -2)
  line L8 (104, -2) -> (-104, -2)
  line L9 (-104, -2) -> (-104, -19)
  line L10 (-104, -19) -> (-106, -19)
  line L11 (-106, -19) -> (-106, -9)
  line L12 (-106, -17) -> (-107.5, -12.2)
  line L13 (-107.5, -12.2) -> (-106, -12.2)
  line L14 (-106, -17) -> (-106, -12.2)
  line L15 (0, -20) -> (0, -2.5)
  line L16 (106, -19) -> (106, -9)
  line L17 (107.5, -12.2) -> (106, -12.2)
  line L18 (106, -17) -> (106, -12.2)
  line L19 (104, -19) -> (106, -19)
  line L20 (106, -17) -> (107.5, -12.2)
  line L21 (106, -9) -> (108, -9)
  dimension "d77" = 1.5
  dimension "d78" = 4.8
  dimension "d79" = 2
  constraint coincident L11 L12.start
  constraint coincident L11 L13.end
  constraint perpendicular L11 L13
  constraint symmetric L0.start L15 L4.end
  constraint symmetric L0.end L15 L3.end
  constraint symmetric L9.end L15 L6.end
  constraint symmetric L10.end L15 L5.end
  constraint symmetric L12.start L15 L18.start
  constraint symmetric L12.end L15 L17.start
  constraint symmetric L13.end L15 L17.end
  measures "d77" distance of L12.end L13.end
  measures "d78" distance of L12.start L13
  measures "d79" distance of L10 L12.start
extrude "押し出し6" add sketch "スケッチ7" along normal mid plane 12 contours L11 L12 L13 L14 | L5 L16 L17 L18 L20